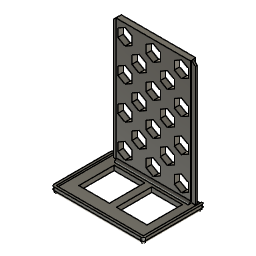
DFRobotWeatherBH4TDV v4 (Autodesk Fusion 360 archive; units mm, degrees)
design "DFRobotWeatherLid"
Autodesk Fusion 360 part; units mm, degrees
sketch "Sketch1" plane through (0, 0, 0) normal (0, 0, 1) x (1, 0, 0)
  line L0 (0, 0) -> (39, 0)
  line L1 (39, 0) -> (39, 26)
  line L2 (39, 26) -> (0, 26)
  line L3 (0, 26) -> (0, 0)
  line L4 (0, 6.6) -> (39, 6.6) construction
  line L5 (19.5, 26) -> (19.5, 0) construction
  line L6 (18, 6.6) -> (5, 6.6)
  line L7 (5, 6.6) -> (5, 21.6)
  line L8 (5, 21.6) -> (18, 21.6)
  line L9 (18, 21.6) -> (18, 6.6)
  line L10 (21, 21.6) -> (21, 6.6)
  line L11 (21, 6.6) -> (34, 6.6)
  line L12 (34, 6.6) -> (34, 21.6)
  line L13 (34, 21.6) -> (21, 21.6)
  dimension "d1" = 39
  dimension "d2" = 26
  dimension "d3" = 13
  dimension "d4" = 15
  dimension "d5" = 1.5
  dimension "d6" = 6.6
  constraint horizontal L0
  constraint vertical L1
  constraint horizontal L2
  constraint vertical L3
  constraint coincident L0.start L3.end
  constraint coincident L3 L4.start
  constraint coincident L1 L4.end
  constraint perpendicular L1 L4
  constraint midpoint L2 L5.start
  constraint midpoint L0 L5.end
  constraint horizontal L6
  constraint vertical L7
  constraint horizontal L8
  constraint vertical L9
  constraint collinear L4 L6
  constraint symmetric L5 L6.start L10.end
  constraint symmetric L5 L6.end L11.end
  constraint symmetric L5 L7.end L12.end
  constraint symmetric L5 L8.end L10.start
  measures "d1" distance of L0.start L0.end
  measures "d2" distance of L0.start L2.end
  measures "d3" distance of L6.start L6.end
  measures "d4" distance of L6.start L8.end
  measures "d5" distance of L5 L9
  measures "d6" distance of L0 L4
extrude "Extrude1" add sketch "Sketch1" along normal blind 2
sketch "Sketch2" plane through (0, 0, 2) normal (0, 0, 1) x (-1, 0, 0)
  line L0 (-21, -21.6) -> (-34, -21.6)
  line L1 (-34, -21.6) -> (-34, -6.6)
  line L2 (-34, -6.6) -> (-21, -6.6)
  line L3 (-21, -6.6) -> (-21, -21.6)
  line L4 (-5, -21.6) -> (-18, -21.6)
  line L5 (-18, -21.6) -> (-18, -6.6)
  line L6 (-18, -6.6) -> (-5, -6.6)
  line L7 (-5, -6.6) -> (-5, -21.6)
  line L8 (0, -26) -> (0, 0)
  line L9 (0, 0) -> (-39, 0)
  line L10 (-39, 0) -> (-39, -26)
  line L11 (-39, -26) -> (0, -26)
  line L12 (-3.7, -26) -> (-3.7, -25)
  line L13 (-3.7, -25) -> (-2.1, -25)
  line L14 (-2.1, -24.2) -> (-3.7, -24.2)
  line L15 (-3.7, -24.2) -> (-3.7, -23.7)
  line L16 (-19.5, -26) -> (-19.5, 0) construction
  line L17 (-2.1, -25) -> (-2.1, -24.2)
  line L18 (-35.3, -26) -> (-35.3, -25)
  line L19 (-35.3, -25) -> (-39, -25)
  line L20 (-39, -25) -> (-39, -24.2)
  line L21 (-39, -24.2) -> (-35.3, -24.2)
  line L22 (-35.3, -24.2) -> (-35.3, -23.7)
  line L23 (-3.7, -23.7) -> (-35.3, -23.7)
  line L24 (-3.7, -26) -> (-35.3, -26)
  line L25 (-36.9, -24.2) -> (-35.3, -24.2)
  line L26 (-36.9, -25) -> (-36.9, -24.2)
  line L27 (-35.3, -25) -> (-36.9, -25)
  dimension "d9" = 3.7
  dimension "d10" = 1
  dimension "d11" = 0.8
  dimension "d12" = 0.5
  dimension "d45" = 1.6
  dimension "d46" = 2.1
  constraint coincident L11 L12.start
  constraint perpendicular L11 L12
  constraint perpendicular L12 L13
  constraint perpendicular L8 L14
  constraint perpendicular L14 L15
  constraint midpoint L11 L16.start
  constraint midpoint L9 L16.end
  constraint symmetric L12.start L16 L18.start
  constraint symmetric L12.end L16 L18.end
  constraint symmetric L14.end L16 L21.end
  constraint symmetric L15.end L16 L22.end
  constraint symmetric L16 L13.end L26.start
  constraint symmetric L16 L14.start L25.start
  measures "d9" distance of L8.start L12.start
  measures "d10" distance of L12.start L12.end
  measures "d11" distance of L13 L14.start
  measures "d12" distance of L14.end L15.end
  measures "d45" distance of L14.end L14.start
  measures "d46" distance of L8 L17
extrude "Extrude2" add sketch "Sketch2" along normal blind 52.5 contours L11 L12 L13 L14 L15 L17 L18 L19 L21 L22 L23 L24 L25 L26 L27
sketch "Sketch3" plane through (0, 0, 2) normal (0, 0, 1) x (-1, 0, 0)
  line L0 (-5, -21.6) -> (-18, -21.6)
  line L1 (-18, -21.6) -> (-18, -6.6)
  line L2 (-18, -6.6) -> (-5, -6.6)
  line L3 (-5, -6.6) -> (-5, -21.6)
  line L4 (-21, -21.6) -> (-34, -21.6)
  line L5 (-34, -21.6) -> (-34, -6.6)
  line L6 (-34, -6.6) -> (-21, -6.6)
  line L7 (-21, -6.6) -> (-21, -21.6)
  line L8 (-36.9, -24.2) -> (-35.3, -24.2)
  line L9 (-35.3, -24.2) -> (-35.3, -23.7)
  line L10 (-35.3, -23.7) -> (-3.7, -23.7)
  line L11 (-3.7, -23.7) -> (-3.7, -24.2)
  line L12 (-3.7, -24.2) -> (-2.1, -24.2)
  line L13 (-2.1, -24.2) -> (-2.1, -25)
  line L14 (0, 0) -> (-39, 0)
  line L15 (-39, 0) -> (-39, -26)
  line L16 (-38, -1) -> (-38, -22.7)
  line L17 (-1, -22.7) -> (-1, -1)
  line L18 (-1, -1) -> (-38, -1)
  line L19 (-38, -22.7) -> (-38, -24.2)
  line L20 (-1, -22.7) -> (-1, -24.2)
  line L21 (-2.1, -25) -> (-3.7, -25)
  line L22 (-3.7, -25) -> (-3.7, -26)
  line L23 (-3.7, -26) -> (0, -26)
  line L24 (0, -26) -> (0, 0)
  line L25 (-35.3, -26) -> (-35.3, -25)
  line L26 (-35.3, -25) -> (-36.9, -25)
  line L27 (-36.9, -25) -> (-36.9, -24.2)
  line L28 (-39, -26) -> (-35.3, -26)
  line L29 (-1, -24.2) -> (-1, -26)
  line L30 (-38, -24.2) -> (-38, -26)
  constraint parallel L15 L16
  constraint parallel L13 L17
  constraint parallel L14 L18
  constraint vertical L19
  constraint coincident L8 L19.end
  constraint vertical L20
  constraint coincident L12 L20.end
  constraint coincident L23 L29.end
  constraint perpendicular L23 L29
  constraint coincident L28 L30.end
  constraint perpendicular L28 L30
extrude "Extrude3" add sketch "Sketch3" along normal blind 0.8 contours L14 L15 L16 L17 L18 L19 L20 L23 L24 L28 L29 L30
sketch "Sketch4" plane through (0, 26, 0) normal (0, 1, 0) x (-1, 0, 0)
  line L0 (-39, 0) -> (0, 0)
  line L1 (0, 0) -> (0, 2.8)
  line L2 (-3.7, 2) -> (-3.7, 54.5)
  line L3 (-3.7, 54.5) -> (-35.3, 54.5)
  line L4 (-35.3, 54.5) -> (-35.3, 2)
  line L5 (-39, 2.8) -> (-39, 0)
  line L6 (-19.5, 54.5) -> (-19.5, 0) construction
  line L7 (-28.5, 51.2321) -> (-31.5, 52.9641)
  line L8 (-31.5, 52.9641) -> (-34.5, 51.2321)
  line L9 (-34.5, 51.2321) -> (-34.5, 47.7679)
  line L10 (-34.5, 47.7679) -> (-31.5, 46.0359)
  line L11 (-31.5, 46.0359) -> (-28.5, 47.7679)
  line L12 (-28.5, 47.7679) -> (-28.5, 51.2321)
  line L13 (-22.5, 51.2321) -> (-22.5, 47.7679)
  line L14 (-22.5, 47.7679) -> (-19.5, 46.0359)
  line L15 (-19.5, 46.0359) -> (-16.5, 47.7679)
  line L16 (-16.5, 47.7679) -> (-16.5, 51.2321)
  line L17 (-16.5, 51.2321) -> (-19.5, 52.9641)
  line L18 (-19.5, 52.9641) -> (-22.5, 51.2321)
  line L19 (-10.5, 51.2321) -> (-10.5, 47.7679)
  line L20 (-10.5, 47.7679) -> (-7.5, 46.0359)
  line L21 (-7.5, 46.0359) -> (-4.5, 47.7679)
  line L22 (-4.5, 47.7679) -> (-4.5, 51.2321)
  line L23 (-4.5, 51.2321) -> (-7.5, 52.9641)
  line L24 (-7.5, 52.9641) -> (-10.5, 51.2321)
  line L25 (-22.5, 44.3038) -> (-25.5, 46.0359)
  line L26 (-25.5, 46.0359) -> (-28.5, 44.3038)
  line L27 (-28.5, 44.3038) -> (-28.5, 40.8397)
  line L28 (-28.5, 40.8397) -> (-25.5, 39.1077)
  line L29 (-25.5, 39.1077) -> (-22.5, 40.8397)
  line L30 (-22.5, 40.8397) -> (-22.5, 44.3038)
  line L31 (-10.5, 44.3038) -> (-13.5, 46.0359)
  line L32 (-13.5, 46.0359) -> (-16.5, 44.3038)
  line L33 (-16.5, 44.3038) -> (-16.5, 40.8397)
  line L34 (-16.5, 40.8397) -> (-13.5, 39.1077)
  line L35 (-13.5, 39.1077) -> (-10.5, 40.8397)
  line L36 (-10.5, 40.8397) -> (-10.5, 44.3038)
  line L37 (-34.5, 37.2321) -> (-34.5, 33.7679)
  line L38 (-34.5, 33.7679) -> (-31.5, 32.0359)
  line L39 (-31.5, 32.0359) -> (-28.5, 33.7679)
  line L40 (-28.5, 33.7679) -> (-28.5, 37.2321)
  line L41 (-28.5, 37.2321) -> (-31.5, 38.9641)
  line L42 (-31.5, 38.9641) -> (-34.5, 37.2321)
  line L43 (-28.5, 30.3038) -> (-28.5, 26.8397)
  line L44 (-28.5, 26.8397) -> (-25.5, 25.1077)
  line L45 (-25.5, 25.1077) -> (-22.5, 26.8397)
  line L46 (-22.5, 26.8397) -> (-22.5, 30.3038)
  line L47 (-25.5, 32.0359) -> (-28.5, 30.3038)
  line L48 (-22.5, 30.3038) -> (-25.5, 32.0359)
  line L49 (-22.5, 37.2321) -> (-22.5, 33.7679)
  line L50 (-22.5, 33.7679) -> (-19.5, 32.0359)
  line L51 (-19.5, 32.0359) -> (-16.5, 33.7679)
  line L52 (-16.5, 33.7679) -> (-16.5, 37.2321)
  line L53 (-19.5, 38.9641) -> (-22.5, 37.2321)
  line L54 (-16.5, 37.2321) -> (-19.5, 38.9641)
  line L55 (-16.5, 26.8397) -> (-13.5, 25.1077)
  line L56 (-13.5, 25.1077) -> (-10.5, 26.8397)
  line L57 (-10.5, 26.8397) -> (-10.5, 30.3038)
  line L58 (-10.5, 30.3038) -> (-13.5, 32.0359)
  line L59 (-16.5, 30.3038) -> (-16.5, 26.8397)
  line L60 (-13.5, 32.0359) -> (-16.5, 30.3038)
  line L61 (-4.5, 33.7679) -> (-4.5, 37.2321)
  line L62 (-4.5, 37.2321) -> (-7.5, 38.9641)
  line L63 (-7.5, 38.9641) -> (-10.5, 37.2321)
  line L64 (-10.5, 37.2321) -> (-10.5, 33.7679)
  line L65 (-7.5, 32.0359) -> (-4.5, 33.7679)
  line L66 (-10.5, 33.7679) -> (-7.5, 32.0359)
  line L67 (-34.5, 23.2321) -> (-34.5, 19.7679)
  line L68 (-34.5, 19.7679) -> (-31.5, 18.0359)
  line L69 (-31.5, 18.0359) -> (-28.5, 19.7679)
  line L70 (-28.5, 19.7679) -> (-28.5, 23.2321)
  line L71 (-28.5, 23.2321) -> (-31.5, 24.9641)
  line L72 (-31.5, 24.9641) -> (-34.5, 23.2321)
  line L73 (-28.5, 16.3038) -> (-28.5, 12.8397)
  line L74 (-28.5, 12.8397) -> (-25.5, 11.1077)
  line L75 (-25.5, 11.1077) -> (-22.5, 12.8397)
  line L76 (-22.5, 12.8397) -> (-22.5, 16.3038)
  line L77 (-25.5, 18.0359) -> (-28.5, 16.3038)
  line L78 (-22.5, 16.3038) -> (-25.5, 18.0359)
  line L79 (-22.5, 23.2321) -> (-22.5, 19.7679)
  line L80 (-22.5, 19.7679) -> (-19.5, 18.0359)
  line L81 (-19.5, 18.0359) -> (-16.5, 19.7679)
  line L82 (-16.5, 19.7679) -> (-16.5, 23.2321)
  line L83 (-19.5, 24.9641) -> (-22.5, 23.2321)
  line L84 (-16.5, 23.2321) -> (-19.5, 24.9641)
  line L85 (-16.5, 12.8397) -> (-13.5, 11.1077)
  line L86 (-13.5, 11.1077) -> (-10.5, 12.8397)
  line L87 (-10.5, 12.8397) -> (-10.5, 16.3038)
  line L88 (-10.5, 16.3038) -> (-13.5, 18.0359)
  line L89 (-16.5, 16.3038) -> (-16.5, 12.8397)
  line L90 (-13.5, 18.0359) -> (-16.5, 16.3038)
  line L91 (-4.5, 19.7679) -> (-4.5, 23.2321)
  line L92 (-4.5, 23.2321) -> (-7.5, 24.9641)
  line L93 (-7.5, 24.9641) -> (-10.5, 23.2321)
  line L94 (-10.5, 23.2321) -> (-10.5, 19.7679)
  line L95 (-7.5, 18.0359) -> (-4.5, 19.7679)
  line L96 (-10.5, 19.7679) -> (-7.5, 18.0359)
  line L97 (-34.5, 9.2321) -> (-34.5, 5.7679)
  line L98 (-34.5, 5.7679) -> (-31.5, 4.0359)
  line L99 (-31.5, 4.0359) -> (-28.5, 5.7679)
  line L100 (-28.5, 5.7679) -> (-28.5, 9.2321)
  line L101 (-28.5, 9.2321) -> (-31.5, 10.9641)
  line L102 (-31.5, 10.9641) -> (-34.5, 9.2321)
  line L103 (-22.5, 9.2321) -> (-22.5, 5.7679)
  line L104 (-22.5, 5.7679) -> (-19.5, 4.0359)
  line L105 (-19.5, 4.0359) -> (-16.5, 5.7679)
  line L106 (-16.5, 5.7679) -> (-16.5, 9.2321)
  line L107 (-19.5, 10.9641) -> (-22.5, 9.2321)
  line L108 (-16.5, 9.2321) -> (-19.5, 10.9641)
  line L109 (-4.5, 5.7679) -> (-4.5, 9.2321)
  line L110 (-4.5, 9.2321) -> (-7.5, 10.9641)
  line L111 (-7.5, 10.9641) -> (-10.5, 9.2321)
  line L112 (-10.5, 9.2321) -> (-10.5, 5.7679)
  line L113 (-7.5, 4.0359) -> (-4.5, 5.7679)
  line L114 (-10.5, 5.7679) -> (-7.5, 4.0359)
  line L115 (0, 2.8) -> (-1, 2.8)
  line L116 (-38, 2.8) -> (-39, 2.8)
  line L117 (-1, 2.8) -> (-1, 2)
  line L118 (-1, 2) -> (-3.7, 2)
  line L119 (-35.3, 2) -> (-38, 2)
  line L120 (-38, 2) -> (-38, 2.8)
  point P0 (-31.5, 49.5)
  point P1 (-25.5, 42.5718)
  dimension "d18" = 3
  dimension "d19" = 5
  dimension "d20" = 90
  dimension "d21" = 0.8
  dimension "d24" = 12
  dimension "d25" = 0
  dimension "d26" = 3
  dimension "d27" = 90
  dimension "d28" = 3
  dimension "d29" = 3
  dimension "d32" = 12
  dimension "d33" = 0
  dimension "d36" = 0
  dimension "d37" = -14
  constraint midpoint L3 L6.start
  constraint midpoint L0 L6.end
  measures "d18" distance of P0 L12
  measures "d19" distance of L3 P0
  measures "d20" angle of L3 L9
  measures "d21" distance of L4 L9
  measures "d26" distance of P1 L30
  measures "d27" angle of L3 L27
  measures "d28" distance of L14 L25
  measures "d29" distance of L11 L26
extrude "Extrude4" cut sketch "Sketch4" against normal blind 3 contours L7 L8 L9 L10 L11 L12 | L13 L14 L15 L16 L17 L18 | L19 L20 L21 L22 L23 L24 | L25 L26 L27 L28 L29 L30 | L31 L32 L33 L34 L35 L36 | L37 L38 L39 L40 L41 L42 | L43 L44 L45 L46 L47 L48 | L49 L50 L51 L52 L53 L54 | L55 L56 L57 L58 L59 L60 | L61 L62 L63 L64 L65 L66 | L67 L68 L69 L70 L71 L72 | L73 L74 L75 L76 L77 L78 | L79 L80 L81 L82 L83 L84 | L85 L86 L87 L88 L89 L90 | L91 L92 L93 L94 L95 L96 | L97 L98 L99 L100 L101 L102 | L103 L104 L105 L106 L107 L108 | L109 L110 L111 L112 L113 L114
fillet "Fillet1" radius 1 1 edges at (19.5, 23.7, 2)
fillet "Fillet3" radius 1 4 edges at (39, 26, 1.4) (39, 0, 1.4) (0, 26, 1.4) (0, 0, 1.4)
fillet "Fillet2" radius 1.5 3 edges at (39, 13, 0) (19.5, 26, 0) (0, 13, 0)
chamfer "Chamfer1" distance 1.5 angle 45 1 edges at (2.1, 24.6, 54.5)
chamfer "Chamfer1" distance 1.5 angle 45 1 edges at (36.9, 24.6, 54.5)
equation "d6 = 2 mm + 3 mm + 1.6 mm"
